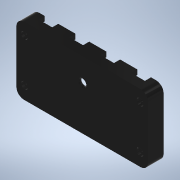
# Autodesk Inventor part: casing-top
Saved by Autodesk Inventor 2021 (Build 250183000, 183)
## iProperties
Created: 2022-04-04
Part Number: casing-top
Material: PET Plastic
Document SubType Name: Modeling
Designer: Staňa
Density: 1.541 g/cm^3
Appearance: Smooth - Black
Author: Staňa
Autodesk Inventor part; units mm, degrees
ref_plane "YZ Plane" through (0, 0, 0) normal (1, 0, 0) x (0, 1, 0)
ref_plane "XZ Plane" through (0, 0, 0) normal (0, 1, 0) x (-1, 0, 0)
ref_plane "XY Plane" through (0, 0, 0) normal (0, 0, 1) x (1, 0, 0)
sketch "Sketch2" plane through (0, 0, 0) normal (0, 0, 1) x (1, 0, 0)
  arc A0 (-53.25, -24.2999) -> (-47.25, -30.2999) centre (-47.25, -24.2999) ccw projected
  line L0 (-47.25, -30.2999) -> (47.25, -30.2999) projected
  arc A1 (47.25, -30.2999) -> (53.25, -24.2999) centre (47.25, -24.2999) ccw projected
  line L1 (53.25, -24.2999) -> (53.25, 18.2499) projected
  arc A2 (53.25, 18.2499) -> (47.25, 24.2499) centre (47.25, 18.2499) ccw projected
  line L2 (47.25, 24.2499) -> (-47.25, 24.2499) projected
  arc A3 (-47.25, 24.2499) -> (-53.25, 18.2499) centre (-47.25, 18.2499) ccw projected
  line L3 (-53.25, 18.2499) -> (-53.25, -24.2999) projected
  line L4 (-6.9201, 18.5) -> (-6.9201, 20) construction
  line L5 (-6.9201, 20) -> (6.9199, 20) projected
  line L6 (6.9199, 20) -> (6.9199, 18.5) construction
  line L7 (6.9199, 18.5) -> (18.0799, 18.5) construction
  line L8 (18.0799, 18.5) -> (18.0799, 20) construction
  line L9 (18.0799, 20) -> (31.9199, 20) projected
  line L10 (31.9199, 20) -> (31.9199, 18.5) construction
  line L11 (31.9199, 18.5) -> (43.0799, 18.5) construction
  line L12 (43.0799, 18.5) -> (43.0799, 20) construction
  line L13 (43.0799, 20) -> (46.7497, 20) projected
  arc A4 (51.75, 14.9997) -> (46.7497, 20) centre (46.7497, 14.9997) ccw projected
  line L14 (51.75, 14.9997) -> (51.75, -19.9997) projected
  arc A5 (46.7497, -25) -> (51.75, -19.9997) centre (46.7497, -19.9997) ccw projected
  line L15 (46.7497, -25) -> (35.8301, -25) projected
  line L16 (35.8301, -25) -> (35.8301, -23.5) construction
  line L17 (35.8301, -23.5) -> (-35.8299, -23.5) construction
  line L18 (-35.8299, -23.5) -> (-35.8299, -25) construction
  line L19 (-35.8299, -25) -> (-46.7497, -25) projected
  arc A6 (-51.75, -19.9997) -> (-46.7497, -25) centre (-46.7497, -19.9997) ccw projected
  line L20 (-51.75, -19.9997) -> (-51.75, 14.9997) projected
  arc A7 (-46.7497, 20) -> (-51.75, 14.9997) centre (-46.7497, 14.9997) ccw projected
  line L21 (-46.7497, 20) -> (-43.0801, 20) projected
  line L22 (-43.0801, 20) -> (-43.0801, 18.5) construction
  line L23 (-43.0801, 18.5) -> (-31.9201, 18.5) construction
  line L24 (-31.9201, 18.5) -> (-31.9201, 20) construction
  line L25 (-31.9201, 20) -> (-18.0801, 20) projected
  line L26 (-18.0801, 20) -> (-18.0801, 18.5) construction
  line L27 (-18.0801, 18.5) -> (-6.9201, 18.5) construction
  line L28 (-43.0801, 20) -> (-43.0801, 24.2499)
  line L29 (-31.9201, 20) -> (-31.9201, 24.2499)
  line L30 (-18.0801, 20) -> (-18.0801, 24.2499)
  line L31 (-6.9201, 20) -> (-6.9201, 24.2499)
  line L32 (6.9199, 20) -> (6.9199, 24.2499)
  line L33 (18.0799, 20) -> (18.0799, 24.2499)
  line L34 (31.9199, 20) -> (31.9199, 24.2499)
  line L35 (43.0799, 20) -> (43.0799, 24.2499)
  line L36 (35.8301, -25) -> (35.8301, -30.2999)
  line L37 (-35.8299, -25) -> (-35.8299, -30.2999)
  point P0 (0, 0)
  constraints: 20 end point, 2 perpendicular, 2 point on line, 17 other
extrude "Extrusion3" add sketch "Sketch2" along normal blind 5.2 contours L3 A3 L2 L28 L21 A7 L20 A6 L19 L37 L0 A0 | L36 L15 A5 L14 A4 L13 L35 L2 A2 L1 A1 L0 | L2 L30 L25 L29 | L2 L32 L5 L31 | L2 L34 L9 L33
ref_plane "Work Plane1" through (-43.79, -2.5, 1.5) normal (0, 0, 1) x (1, 0, 0)
sketch "Sketch3" plane through (-43.79, -2.5, 1.5) normal (0, 0, 1) x (1, 0, 0)
  line L0 (-6.46, -17.4997) -> (-6.46, 17.4997) projected
  arc A0 (-2.9597, 21) -> (-6.46, 17.4997) centre (-2.9597, 17.4997) ccw projected
  line L1 (-2.9597, 21) -> (0.7099, 21) projected
  line L2 (0.7099, 21) -> (0.7099, 22.5) projected
  line L3 (0.7099, 22.5) -> (-2.9597, 22.5) projected
  arc A1 (-2.9597, 22.5) -> (-7.96, 17.4997) centre (-2.9597, 17.4997) ccw projected
  line L4 (-7.96, 17.4997) -> (-7.96, -17.4997) projected
  arc A2 (-7.96, -17.4997) -> (-2.9597, -22.5) centre (-2.9597, -17.4997) ccw projected
  line L5 (-2.9597, -22.5) -> (7.96, -22.5) projected
  line L6 (7.96, -22.5) -> (7.96, -21) projected
  line L7 (7.96, -21) -> (-2.9597, -21) projected
  arc A3 (-6.46, -17.4997) -> (-2.9597, -21) centre (-2.9597, -17.4997) ccw projected
  line L8 (25.7099, 22.5) -> (11.8699, 22.5) projected
  line L9 (11.8699, 22.5) -> (11.8699, 21) projected
  line L10 (11.8699, 21) -> (25.7099, 21) projected
  line L11 (25.7099, 21) -> (25.7099, 22.5) projected
  line L12 (50.7099, 22.5) -> (36.8699, 22.5) projected
  line L13 (36.8699, 22.5) -> (36.8699, 21) projected
  line L14 (36.8699, 21) -> (50.7099, 21) projected
  line L15 (50.7099, 21) -> (50.7099, 22.5) projected
  line L16 (75.7099, 22.5) -> (61.8699, 22.5) projected
  line L17 (61.8699, 22.5) -> (61.8699, 21) projected
  line L18 (61.8699, 21) -> (75.7099, 21) projected
  line L19 (75.7099, 21) -> (75.7099, 22.5) projected
  line L20 (90.5396, -21) -> (79.62, -21) projected
  line L21 (79.62, -21) -> (79.62, -22.5) projected
  line L22 (79.62, -22.5) -> (90.5396, -22.5) projected
  arc A4 (90.5396, -22.5) -> (95.54, -17.4997) centre (90.5396, -17.4997) ccw projected
  line L23 (95.54, -17.4997) -> (95.54, 17.4997) projected
  arc A5 (95.54, 17.4997) -> (90.5396, 22.5) centre (90.5396, 17.4997) ccw projected
  line L24 (90.5396, 22.5) -> (86.8699, 22.5) projected
  line L25 (86.8699, 22.5) -> (86.8699, 21) projected
  line L26 (86.8699, 21) -> (90.5396, 21) projected
  arc A6 (94.04, 17.4997) -> (90.5396, 21) centre (90.5396, 17.4997) ccw projected
  line L27 (94.04, 17.4997) -> (94.04, -17.4997) projected
  arc A7 (90.5396, -21) -> (94.04, -17.4997) centre (90.5396, -17.4997) ccw projected
  point P0 (43.79, 2.5)
  point P1 (90.5396, 22.5)
  point P2 (-2.9597, 21)
  point P3 (-7.96, 17.4997)
  point P4 (-2.9597, -21)
extrude "Extrusion4" add sketch "Sketch3" along normal up to surface (3.7 mm away)
thicken "Thicken1" operation add thickness 0.25 both sides no extend neighbours yes toward (-1, 0, 0) faces at (-51.75, 3.3332, 1) (-48.5765, 19.6543, 0.5) (-45.5265, 20, 0.5) (-50.1508, -23.6652, 0.5) (-39.4698, -25, 0.5) (-52.75, -8.6832, 0)
thicken "Thicken2" operation add thickness 0.25 both sides no extend neighbours yes toward (0, 1, 0) faces at (-27.3068, 20, 1) (-22.6934, 21.4166, 0)
thicken "Thicken3" operation add thickness 0.25 both sides no extend neighbours yes toward (0, 1, 0) faces at (-2.3068, 20, 1) (2.3066, 21.4166, 0)
thicken "Thicken4" operation add thickness 0.25 both sides no extend neighbours yes toward (0, 1, 0) faces at (22.6932, 20, 1) (27.3066, 21.4166, 0)
thicken "Thicken5" operation add thickness 0.25 both sides no extend neighbours yes toward (0, 1, 0) faces at (44.3032, 20, 1) (49.5665, 19.1311, 1) (51.75, 3.3332, 0.5) (47.4949, -24.9442, 1) (43.1098, -25, 1) (52.75, -8.6832, 0)
sketch "Sketch4" plane through (0, 0, 0) normal (0, 0, 1) x (1, 0, 0)
  line L0 (-47.25, -30.2999) -> (-35.8299, -30.2999) projected
  line L1 (-35.8299, -30.2999) -> (-35.8299, -23.5) projected
  line L2 (-46.7497, -23.5) -> (-35.8299, -23.5) projected
  arc A0 (-50.25, -19.9997) -> (-46.7497, -23.5) centre (-46.7497, -19.9997) ccw projected
  line L3 (-50.25, 14.9997) -> (-50.25, -19.9997) projected
  arc A1 (-46.7497, 18.5) -> (-50.25, 14.9997) centre (-46.7497, 14.9997) ccw projected
  line L4 (-43.0801, 18.5) -> (-46.7497, 18.5) projected
  line L5 (-43.0801, 24.2499) -> (-43.0801, 18.5) construction
  line L6 (-43.0801, 24.2499) -> (-47.25, 24.2499) projected
  arc A2 (-47.25, 24.2499) -> (-53.25, 18.2499) centre (-47.25, 18.2499) ccw projected
  line L7 (-53.25, 18.2499) -> (-53.25, -24.2999) projected
  arc A3 (-53.25, -24.2999) -> (-47.25, -30.2999) centre (-47.25, -24.2999) ccw projected
  line L8 (-18.0801, 24.2499) -> (-18.0801, 18.5) construction
  line L9 (-18.0801, 24.2499) -> (-31.9201, 24.2499) projected
  line L10 (-31.9201, 24.2499) -> (-31.9201, 18.5) construction
  line L11 (-18.0801, 18.5) -> (-31.9201, 18.5) projected
  line L12 (6.9199, 24.2499) -> (6.9199, 18.5) construction
  line L13 (6.9199, 24.2499) -> (-6.9201, 24.2499) projected
  line L14 (-6.9201, 24.2499) -> (-6.9201, 18.5) construction
  line L15 (6.9199, 18.5) -> (-6.9201, 18.5) projected
  line L16 (31.9199, 24.2499) -> (31.9199, 18.5) construction
  line L17 (31.9199, 24.2499) -> (18.0799, 24.2499) projected
  line L18 (18.0799, 24.2499) -> (18.0799, 18.5) construction
  line L19 (31.9199, 18.5) -> (18.0799, 18.5) projected
  line L20 (47.25, 24.2499) -> (43.0799, 24.2499) projected
  line L21 (43.0799, 24.2499) -> (43.0799, 18.5) construction
  line L22 (46.7497, 18.5) -> (43.0799, 18.5) projected
  arc A4 (50.25, 14.9997) -> (46.7497, 18.5) centre (46.7497, 14.9997) ccw projected
  line L23 (50.25, -19.9997) -> (50.25, 14.9997) projected
  arc A5 (46.7497, -23.5) -> (50.25, -19.9997) centre (46.7497, -19.9997) ccw projected
  line L24 (35.8301, -23.5) -> (46.7497, -23.5) projected
  line L25 (35.8301, -30.2999) -> (35.8301, -23.5) projected
  line L26 (35.8301, -30.2999) -> (47.25, -30.2999) projected
  arc A6 (47.25, -30.2999) -> (53.25, -24.2999) centre (47.25, -24.2999) ccw projected
  line L27 (53.25, -24.2999) -> (53.25, 18.2499) projected
  arc A7 (53.25, 18.2499) -> (47.25, 24.2499) centre (47.25, 18.2499) ccw projected
  line L28 (-43.0801, 18.5) -> (-31.9201, 18.5)
  line L29 (-18.0801, 18.5) -> (-6.9201, 18.5)
  line L30 (6.9199, 18.5) -> (18.0799, 18.5)
  line L31 (31.9199, 18.5) -> (43.0799, 18.5)
  line L32 (43.0799, 24.2499) -> (31.9199, 24.2499)
  line L33 (18.0799, 24.2499) -> (6.9199, 24.2499)
  line L34 (-6.9201, 24.2499) -> (-18.0801, 24.2499)
  line L35 (-31.9201, 24.2499) -> (-43.0801, 24.2499)
  point P0 (0, 0)
  constraints: 16 end point, 6 collinear, 2 perpendicular
extrude "Extrusion5" add sketch "Sketch4" along normal blind 4.1 from surface at 5.2
sketch "Sketch5" plane through (0, 0, 0) normal (0, 0, 1) x (1, 0, 0)
  line L0 (47.25, -30.2999) -> (35.8301, -30.2999) projected
  arc A0 (47.25, -30.2999) -> (53.25, -24.2999) centre (47.25, -24.2999) ccw projected
  line L1 (53.25, 18.2499) -> (53.25, -24.2999) projected
  arc A1 (53.25, 18.2499) -> (47.25, 24.2499) centre (47.25, 18.2499) ccw projected
  line L2 (-47.25, 24.2499) -> (47.25, 24.2499) projected
  arc A2 (-47.25, 24.2499) -> (-53.25, 18.2499) centre (-47.25, 18.2499) ccw projected
  line L3 (-53.25, -24.2999) -> (-53.25, 18.2499) projected
  arc A3 (-53.25, -24.2999) -> (-47.25, -30.2999) centre (-47.25, -24.2999) ccw projected
  line L4 (-35.8299, -30.2999) -> (-47.25, -30.2999) projected
  line L5 (-35.8299, -23.5) -> (-35.8299, -30.2999) construction
  line L6 (-46.7497, -23.5) -> (-35.8299, -23.5) projected
  arc A4 (-50.25, -19.9997) -> (-46.7497, -23.5) centre (-46.7497, -19.9997) ccw projected
  line L7 (-50.25, 14.9997) -> (-50.25, -19.9997) projected
  arc A5 (-46.7497, 18.5) -> (-50.25, 14.9997) centre (-46.7497, 14.9997) ccw projected
  line L8 (46.7497, 18.5) -> (-46.7497, 18.5) projected
  arc A6 (50.25, 14.9997) -> (46.7497, 18.5) centre (46.7497, 14.9997) ccw projected
  line L9 (50.25, -19.9997) -> (50.25, 14.9997) projected
  arc A7 (46.7497, -23.5) -> (50.25, -19.9997) centre (46.7497, -19.9997) ccw projected
  line L10 (35.8301, -23.5) -> (46.7497, -23.5) projected
  line L11 (35.8301, -30.2999) -> (35.8301, -23.5) construction
  line L12 (-35.8299, -30.2999) -> (35.8301, -30.2999)
  line L13 (35.8301, -23.5) -> (-35.8299, -23.5)
  point P0 (0, 0)
  constraints: 4 end point, 1 collinear, 1 horizontal
extrude "Extrusion6" add sketch "Sketch5" along normal blind 1 from surface at 9.3
sketch "Sketch6" plane through (-47.25, 24.2499, 10.3) normal (0, 0, 1) x (1, 0.0000001, 0)
  arc A0 (0, 0) -> (-6, -6) centre (0, -6) ccw projected
  line L0 (-6, -48.5499) -> (-6, -6) projected
  arc A1 (-6, -48.5499) -> (0, -54.5499) centre (0, -48.5499) ccw projected
  line L1 (94.5, -54.5499) -> (0, -54.5499) projected
  arc A2 (94.5, -54.5499) -> (100.5, -48.5499) centre (94.5, -48.5499) ccw projected
  line L2 (100.5, -6) -> (100.5, -48.5499) projected
  arc A3 (100.5, -6) -> (94.5, 0) centre (94.5, -6) ccw projected
  line L3 (0, 0) -> (94.5, 0) projected
  point P0 (47.25, -24.2499)
extrude "Extrusion7" add sketch "Sketch6" along normal blind 2.5
sketch "Sketch9" plane through (-47.25, 24.2499, 10.3) normal (0, 0, -1) x (-1, -0.0000001, 0)
  arc A0 (-0.5003, -47.7499) -> (3, -44.2496) centre (-0.5003, -44.2496) ccw projected
  line L0 (-6.0007, -47.7499) -> (-0.5003, -47.7499) projected
  arc A1 (-6.0007, -47.7499) -> (-4.0003, -45.7496) centre (-6.0007, -45.7496) ccw projected
  line L1 (-4.0003, -45.7496) -> (-4.0003, -44.2496) projected
  arc A2 (-0.5003, -40.7496) -> (-4.0003, -44.2496) centre (-0.5003, -44.2496) ccw projected
  line L2 (-0.5003, -40.7496) -> (0.9997, -40.7496) projected
  arc A3 (0.9997, -40.7496) -> (3, -38.7493) centre (0.9997, -38.7493) ccw projected
  line L3 (3, -44.2496) -> (3, -38.7493) projected
  arc A4 (3, -9.2503) -> (-0.5003, -5.7499) centre (-0.5003, -9.2503) ccw projected
  line L4 (3, -14.7506) -> (3, -9.2503) projected
  arc A5 (3, -14.7506) -> (0.9997, -12.7503) centre (0.9997, -14.7506) ccw projected
  line L5 (0.9997, -12.7503) -> (-0.5003, -12.7503) projected
  arc A6 (-4.0003, -9.2503) -> (-0.5003, -12.7503) centre (-0.5003, -9.2503) ccw projected
  line L6 (-4.0003, -9.2503) -> (-4.0003, -7.7503) projected
  arc A7 (-4.0003, -7.7503) -> (-6.0007, -5.7499) centre (-6.0007, -7.7503) ccw projected
  line L7 (-0.5003, -5.7499) -> (-6.0007, -5.7499) projected
  arc A8 (-93.9997, -5.7499) -> (-97.5, -9.2503) centre (-93.9997, -9.2503) ccw projected
  line L8 (-88.4993, -5.7499) -> (-93.9997, -5.7499) projected
  arc A9 (-88.4993, -5.7499) -> (-90.4997, -7.7503) centre (-88.4993, -7.7503) ccw projected
  line L9 (-90.4997, -7.7503) -> (-90.4997, -9.2503) projected
  arc A10 (-93.9997, -12.7503) -> (-90.4997, -9.2503) centre (-93.9997, -9.2503) ccw projected
  line L10 (-93.9997, -12.7503) -> (-95.4997, -12.7503) projected
  arc A11 (-95.4997, -12.7503) -> (-97.5, -14.7506) centre (-95.4997, -14.7506) ccw projected
  line L11 (-97.5, -9.2503) -> (-97.5, -14.7506) projected
  arc A12 (-97.5, -44.2496) -> (-93.9997, -47.7499) centre (-93.9997, -44.2496) ccw projected
  line L12 (-97.5, -38.7493) -> (-97.5, -44.2496) projected
  arc A13 (-97.5, -38.7493) -> (-95.4997, -40.7496) centre (-95.4997, -38.7493) ccw projected
  line L13 (-95.4997, -40.7496) -> (-93.9997, -40.7496) projected
  arc A14 (-90.4997, -44.2496) -> (-93.9997, -40.7496) centre (-93.9997, -44.2496) ccw projected
  line L14 (-90.4997, -44.2496) -> (-90.4997, -45.7496) projected
  arc A15 (-90.4997, -45.7496) -> (-88.4993, -47.7499) centre (-88.4993, -45.7496) ccw projected
  line L15 (-93.9997, -47.7499) -> (-88.4993, -47.7499) projected
  circle A16 centre (-94, -9.2499) radius 1.7 projected
  circle A17 centre (-94, -44.2499) radius 1.7 projected
  circle A18 centre (-0.5, -44.2499) radius 1.7 projected
  circle A19 centre (-0.5, -9.2499) radius 1.7 projected
  point P0 (-47.25, -24.2499)
  point P1 (3, -9.2503)
  point P2 (-0.5003, -5.7499)
  point P3 (-0.5003, -47.7499)
  point P4 (3, -44.2496)
  point P5 (-93.9997, -5.7499)
  point P6 (-97.5, -9.2503)
extrude "Extrusion9" add sketch "Sketch9" along normal blind 2 contours L0 A1 L1 A2 L2 A3 L3 A0 | L4 A5 L5 A6 L6 A7 L7 A4 | L8 A9 L9 A10 L10 A11 L11 A8 | L12 A13 L13 A14 L14 A15 L15 A12 | A16 | A17 | A18 | A19
sketch "Sketch8" plane through (-47.25, 24.2499, 12.8) normal (0, 0, 1) x (1, 0.0000001, 0)
  circle A0 centre (0.5, -44.2499) radius 1.6 construction
  circle A1 centre (0.5, -9.2499) radius 1.6 construction
  circle A2 centre (94, -9.2499) radius 1.6 construction
  circle A3 centre (94, -44.2499) radius 1.6 construction
  point P0 (47.25, -24.2499)
hole "Hole1" at (-46.75, -20, 12.8) at (-46.75, 15, 12.8) at (46.75, 15, 12.8) at (46.75, -20, 12.8) direction (0, 0, -1) diameter 3.4 end through all counterbore diameter 5.7 counterbore depth 2.2 clearance for "Hex Head Cap Screw ISO 24017" size "M3" standard "ISO"
sketch "Sketch7" plane through (-47.25, 24.2499, 12.8) normal (0, 0, 1) x (1, 0.0000001, 0)
  circle A0 centre (47.2499, -19.2499) radius 2.5 construction
  circle A1 centre (47.2499, -19.2499) radius 2.6
  point P0 (47.25, -24.2499)
  dimension "d26" = 0.1
  constraints: 1 centre point
  measures "d26" radial gap between concentric circles of A0 A1
extrude "Extrusion8" cut sketch "Sketch7" against normal through all
chamfer "Chamfer1" distance 0.75 angle 45 2 edges at (-2.6001, 5, 12.8) (-2.6001, 5, 10.3)
body "Solid3"
